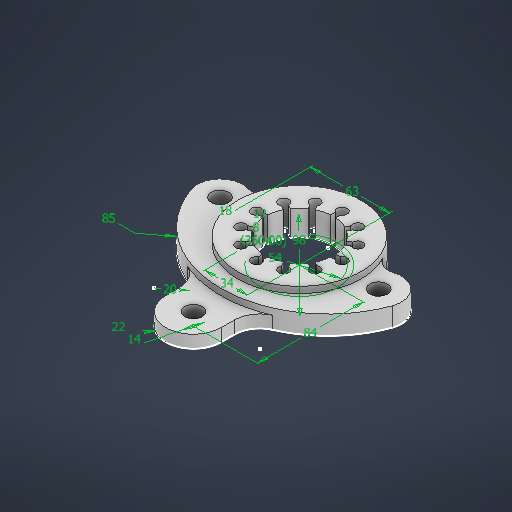
# Autodesk Inventor part: Roseta
Saved by Autodesk Inventor 2026.1 (Build 301233020, 233B)
## iProperties
Created: 2026-02-15
Part Number: Roseta
Material: Generic
Document SubType Name: Modeling
Designer: juanmiguelchungachun
Density: 1 g/cm^3
Appearance: Default
Author: juanmiguelchungachun
Autodesk Inventor part; units mm, degrees
ref_plane "YZ Plane" through (0, 0, 0) normal (1, 0, 0) x (0, 1, 0)
ref_plane "XZ Plane" through (0, 0, 0) normal (0, 1, 0) x (-1, 0, 0)
ref_plane "XY Plane" through (0, 0, 0) normal (0, 0, 1) x (1, 0, 0)
sketch "Sketch1" plane through (0, 0, 0) normal (0, 1, 0) x (-1, 0, 0)
  circle A0 centre (0, 0) radius 7
  arc A1 (22, 0) -> (-22, 0) centre (0, 0) ccw
  line L0 (0, 0) -> (0, -84) construction
  circle A2 centre (0, -84) radius 49
  arc A3 (30.5359, -86) -> (30.5359, -82) centre (34, -84) ccw
  line L1 (26.9258, -82) -> (30.5359, -82)
  line L2 (30.5359, -86) -> (26.9258, -86)
  line L3 (26.9258, -82) -> (30.5359, -86) construction
  line L4 (30.5359, -82) -> (26.9258, -86) construction
  line L5 (27.4449, -70.4641) -> (24.3184, -72.2691)
  arc A4 (27.4449, -70.4641) -> (25.4449, -67) centre (29.4449, -67) ccw
  line L6 (22.3184, -68.805) -> (25.4449, -67)
  line L7 (17, -58.5551) -> (15.195, -61.6816)
  arc A5 (17, -58.5551) -> (13.5359, -56.5551) centre (17, -54.5551) ccw
  line L8 (11.7309, -59.6816) -> (13.5359, -56.5551)
  line L9 (2, -53.4641) -> (2, -57.0742)
  arc A6 (2, -53.4641) -> (-2, -53.4641) centre (0, -50) ccw
  line L10 (-2, -57.0742) -> (-2, -53.4641)
  line L11 (-13.5359, -56.5551) -> (-11.7309, -59.6816)
  arc A7 (-13.5359, -56.5551) -> (-17, -58.5551) centre (-17, -54.5551) ccw
  line L12 (-15.195, -61.6816) -> (-17, -58.5551)
  line L13 (-25.4449, -67) -> (-22.3184, -68.805)
  arc A8 (-25.4449, -67) -> (-27.4449, -70.4641) centre (-29.4449, -67) ccw
  line L14 (-24.3184, -72.2691) -> (-27.4449, -70.4641)
  line L15 (-30.5359, -82) -> (-26.9258, -82)
  arc A9 (-30.5359, -82) -> (-30.5359, -86) centre (-34, -84) ccw
  line L16 (-26.9258, -86) -> (-30.5359, -86)
  line L17 (-27.4449, -97.5359) -> (-24.3184, -95.7309)
  arc A10 (-27.4449, -97.5359) -> (-25.4449, -101) centre (-29.4449, -101) ccw
  line L18 (-22.3184, -99.195) -> (-25.4449, -101)
  line L19 (-17, -109.4449) -> (-15.195, -106.3184)
  arc A11 (-17, -109.4449) -> (-13.5359, -111.4449) centre (-17, -113.4449) ccw
  line L20 (-11.7309, -108.3184) -> (-13.5359, -111.4449)
  line L21 (-2, -114.5359) -> (-2, -110.9258)
  arc A12 (-2, -114.5359) -> (2, -114.5359) centre (0, -118) ccw
  line L22 (2, -110.9258) -> (2, -114.5359)
  line L23 (13.5359, -111.4449) -> (11.7309, -108.3184)
  arc A13 (13.5359, -111.4449) -> (17, -109.4449) centre (17, -113.4449) ccw
  line L24 (15.195, -106.3184) -> (17, -109.4449)
  line L25 (25.4449, -101) -> (22.3184, -99.195)
  arc A14 (25.4449, -101) -> (27.4449, -97.5359) centre (29.4449, -101) ccw
  line L26 (24.3184, -95.7309) -> (27.4449, -97.5359)
  circle A15 centre (63, -84) radius 7
  arc A16 (57.5333, -101.1498) -> (79.9254, -77.8737) centre (63, -84) ccw
  arc A17 (57.5333, -101.1498) -> (43.2878, -106.9601) centre (53.8889, -112.583) ccw
  arc A18 (79.9254, -77.8737) -> (0, -21.8035) centre (0, -106.8035) ccw
  line L27 (22, 0) -> (22, -10.5694)
  arc A19 (22, -10.5694) -> (34, -28.8997) centre (42, -10.5694) ccw
  circle A20 centre (-63, -84) radius 7
  arc A21 (-79.9254, -77.8737) -> (-57.5333, -101.1498) centre (-63, -84) ccw
  arc A22 (-43.2878, -106.9601) -> (-57.5333, -101.1498) centre (-53.8889, -112.583) ccw
  arc A23 (0, -21.8035) -> (-79.9254, -77.8737) centre (0, -106.8035) ccw
  line L28 (-22, 0) -> (-22, -10.5694)
  arc A24 (-34, -28.8997) -> (-22, -10.5694) centre (-42, -10.5694) ccw
  arc A25 (24.3184, -95.7309) -> (26.9258, -86) centre (0, -84) ccw
  arc A26 (15.195, -106.3184) -> (22.3184, -99.195) centre (0, -84) ccw
  arc A27 (2, -110.9258) -> (11.7309, -108.3184) centre (0, -84) ccw
  arc A28 (-11.7309, -108.3184) -> (-2, -110.9258) centre (0, -84) ccw
  arc A29 (-22.3184, -99.195) -> (-15.195, -106.3184) centre (0, -84) ccw
  arc A30 (-26.9258, -86) -> (-24.3184, -95.7309) centre (0, -84) ccw
  arc A31 (-24.3184, -72.2691) -> (-26.9258, -82) centre (0, -84) ccw
  arc A32 (-15.195, -61.6816) -> (-22.3184, -68.805) centre (0, -84) ccw
  arc A33 (-2, -57.0742) -> (-11.7309, -59.6816) centre (0, -84) ccw
  arc A34 (11.7309, -59.6816) -> (2, -57.0742) centre (0, -84) ccw
  arc A35 (26.9258, -82) -> (24.3184, -72.2691) centre (0, -84) ccw
  arc A36 (22.3184, -68.805) -> (15.195, -61.6816) centre (0, -84) ccw
  point P0 (28.7309, -84)
  point P1 (-43.2878, -106.9601)
  dimension "d4" = 98
  dimension "d0" = 14
  dimension "d1" = 22
  dimension "d2" = 84
  dimension "d5" = 8
  dimension "d6" = 34
  dimension "d8" = 4
  dimension "d11" = 360
  dimension "d14" = 63
  dimension "d15" = 18
  dimension "d16" = 12
  dimension "d17" = 85
  dimension "d19" = 20
  dimension "d20" = 54
  constraints: 68 point on circle, 58 end point, 36 centre point, 10 symmetric about line, 6 coincident, 4 horizontal alignment, 4 tangent, 2 midpoint, 2 vertical, 2 vertical alignment, 1 equal radius, 1 horizontal, 1 parallel, 106 other
  measures "d0" diameter of A0
  measures "d1" radius of A1
  measures "d2" distance of L0.start L0.end
  measures "d5" diameter of A3
  measures "d6" distance of A3.centre L0.end
  measures "d8" distance between parallel lines of L2 L1
  measures "d14" distance of A15.centre A25.centre
  measures "d15" radius of A16
  measures "d16" radius of A17
  measures "d17" radius of A18
  measures "d19" radius of A19
  measures "d20" diameter of A35
extrude "Extrusion1" add sketch "Sketch1" along normal blind 10 contours L27 A19 A18 A23 A24 L28 A1
extrude "Extrusion2" add sketch "Sketch1" along normal blind 15 contours A18 A16 A17 A2 A22 A21 A23
extrude "Extrusion3" add sketch "Sketch1" along normal blind 20 contours A2
body "Solid1"
